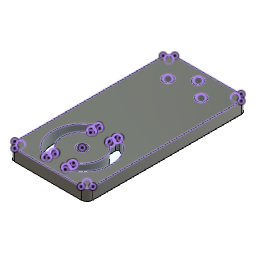
Halterung Kamera BlueFOX v2 (Autodesk Fusion 360 design; units mm, degrees)
Autodesk Fusion 360 part; units mm, degrees
sketch "Skizze1" plane through (0, 0, 0) normal (0, 1, 0) x (1, 0, 0)
  line L0 (0, 0) -> (40, 0)
  line L1 (40, 0) -> (40, 47)
  line L2 (40, 47) -> (0, 47)
  line L3 (0, 47) -> (0, 0)
  circle A0 centre (20, 42) radius 2.5
  circle A1 centre (28.5, 35) radius 2.5
  circle A2 centre (11.5, 35) radius 2.5
  line L4 (0, 0) -> (40, 0)
  line L5 (40, 0) -> (40, -35)
  line L6 (40, -35) -> (0, -35)
  line L7 (0, -35) -> (0, 0)
  circle A3 centre (20, -17.5) radius 15
  circle A4 centre (20, -17.5) radius 10
  line L8 (16, -3.0432) -> (16, -8.3348)
  line L9 (24, -3.0432) -> (24, -8.3348)
  line L10 (16, -26.6652) -> (16, -31.9568)
  line L11 (24, -26.6652) -> (24, -31.9568)
  circle A5 centre (20, -17.5) radius 2.5
  dimension "d1" = 40
  dimension "d2" = 47
  dimension "d3" = 5
  dimension "d4" = 5
  dimension "d5" = 5
  dimension "d6" = 5
  dimension "d7" = 20
  dimension "d8" = 17
  dimension "d9" = 11.5
  dimension "d11" = 7
  dimension "d12" = 30
  dimension "d13" = 20
  dimension "d14" = 17.5
  dimension "d15" = 35
  dimension "d16" = 8
  dimension "d17" = 4
  dimension "d18" = 8
  dimension "d19" = 4
  dimension "d28" = 5
  constraint horizontal L0
  constraint vertical L1
  constraint horizontal L2
  constraint vertical L3
  constraint coincident L0.start L3.end
  constraint horizontal L4
  constraint vertical L5
  constraint horizontal L6
  constraint vertical L7
  constraint concentric A3 A4
  constraint coincident A3 L8.start
  constraint coincident A4 L8.end
  constraint vertical L8
  constraint coincident A3 L9.start
  constraint coincident A4 L9.end
  constraint parallel L8 L9
  constraint coincident A4 L10.start
  constraint coincident A3 L10.end
  constraint parallel L7 L10
  constraint coincident A4 L11.start
  constraint coincident A3 L11.end
  constraint parallel L7 L11
  constraint concentric A3 A5
  measures "d1" distance of L1.end L2.end
  measures "d2" distance of L0.start L2.end
  measures "d3" diameter of A2
  measures "d4" diameter of A0
  measures "d5" diameter of A1
  measures "d6" distance of L2 A0.centre
  measures "d7" distance of L3 A0.centre
  measures "d8" distance of A1.centre A2.centre
  measures "d9" distance of L3 A2.centre
  measures "d11" vertical distance of A0.centre A2.centre
  measures "d12" diameter of A3
  measures "d13" diameter of A4
  measures "d14" distance of L0 A3.centre
  measures "d15" distance of L0.start L6.end
  measures "d16" distance of L8 L9
  measures "d17" distance of A3.centre L8
  measures "d18" distance of L10 L11
  measures "d19" distance of A3.centre L10
  measures "d28" diameter of A5
extrude "Extrusion1" add sketch "Skizze1" along normal blind 6 contours L0 L1 L2 L3 L4 | L0 L4 L5 L6 L7 | A3 A4 L8 L9 | A3 A4 L10 L11 | A4
fillet "Abrundung1" radius 1 4 edges at (24, 3, 3.0432) (24, 3, 26.6652) (24, 3, 8.3348) (24, 3, 31.9568)
fillet "Abrundung1" radius 1 4 edges at (16, 3, 31.9568) (16, 3, 8.3348) (16, 3, 26.6652) (16, 3, 3.0432)
fillet "Abrundung1" radius 3 4 edges at (0, 3, 35) (40, 3, 35) (40, 3, -47) (0, 3, -47)
sketch "Skizze2" plane through (0, 6, 0) normal (0, 1, 0) x (-1, 0, 0)
  arc A0 (-3, -47) -> (0, -44) centre (-3, -44) ccw
  line L0 (0, -44) -> (0, 32)
  arc A1 (0, 32) -> (-3, 35) centre (-3, 32) ccw
  line L1 (-3, 35) -> (-37, 35)
  arc A2 (-37, 35) -> (-40, 32) centre (-37, 32) ccw
  line L2 (-40, 32) -> (-40, -44)
  arc A3 (-40, -44) -> (-37, -47) centre (-37, -44) ccw
  line L3 (-37, -47) -> (-3, -47)
  circle A4 centre (-11.5, -35) radius 2.5
  circle A5 centre (-28.5, -35) radius 2.5
  circle A6 centre (-20, 17.5) radius 2.5
  arc A7 (-14.6429, 3.4893) -> (-14.6429, 31.5107) centre (-20, 17.5) ccw
  arc A8 (-16, 4.4233) -> (-14.6429, 3.4893) centre (-15, 4.4233) ccw
  line L4 (-16, 4.4233) -> (-16, 7.702)
  arc A9 (-15.4545, 8.5928) -> (-16, 7.702) centre (-15, 7.702) ccw
  arc A10 (-15.4545, 8.5928) -> (-15.4545, 26.4072) centre (-20, 17.5) ccw
  arc A11 (-16, 27.298) -> (-15.4545, 26.4072) centre (-15, 27.298) ccw
  line L5 (-16, 27.298) -> (-16, 30.5767)
  arc A12 (-14.6429, 31.5107) -> (-16, 30.5767) centre (-15, 30.5767) ccw
  circle A13 centre (-20, -42) radius 2.5
  line L6 (-24, 30.5767) -> (-24, 27.298)
  arc A14 (-24.5455, 26.4072) -> (-24, 27.298) centre (-25, 27.298) ccw
  arc A15 (-24.5455, 26.4072) -> (-24.5455, 8.5928) centre (-20, 17.5) ccw
  arc A16 (-24, 7.702) -> (-24.5455, 8.5928) centre (-25, 7.702) ccw
  line L7 (-24, 7.702) -> (-24, 4.4233)
  arc A17 (-25.3571, 3.4893) -> (-24, 4.4233) centre (-25, 4.4233) ccw
  arc A18 (-25.3571, 31.5107) -> (-25.3571, 3.4893) centre (-20, 17.5) ccw
  arc A19 (-24, 30.5767) -> (-25.3571, 31.5107) centre (-25, 30.5767) ccw
